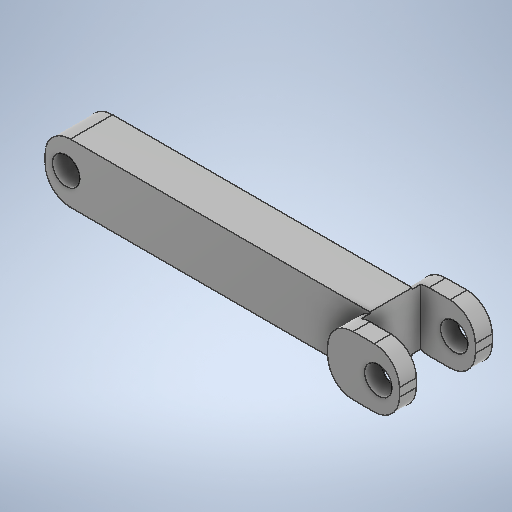
# Autodesk Inventor part: link_arm_1
Saved by Autodesk Inventor 2025 (Build 290162000, 162)
## iProperties
Created: 2025-09-10
Part Number: link_arm_1
Material: 一般
Document SubType Name: Modeling
Designer: sooo1
Density: 1 g/cm^3
Appearance: 滑らか - 標準の灰色
Author: sooo1
Autodesk Inventor part; units mm, degrees
ref_plane "YZ Plane" through (0, 0, 0) normal (1, 0, 0) x (0, 1, 0)
ref_plane "XZ Plane" through (0, 0, 0) normal (0, 1, 0) x (-1, 0, 0)
ref_plane "XY Plane" through (0, 0, 0) normal (0, 0, 1) x (1, 0, 0)
sketch "スケッチ1" plane through (0, 0, 0) normal (0, 0, 1) x (1, 0, 0)
  line L0 (-22.5, 3.5) -> (22.5, 3.5)
  line L1 (22.5, 3.5) -> (22.5, -3.5)
  line L2 (22.5, -3.5) -> (-22.5, -3.5)
  line L3 (-22.5, -3.5) -> (-22.5, 3.5)
  line L4 (-22.5, 3.5) -> (22.5, -3.5) construction
  line L5 (22.5, 3.5) -> (-22.5, -3.5) construction
  line L6 (0, -6.37) -> (0, 6.37) construction
  line L7 (-34.37, 0) -> (34.37, 0) construction
  circle A0 centre (-20, 0) radius 4.55
  line L8 (22.5, -3.5) -> (22.5, 3.5)
  circle A1 centre (20, 0) radius 4.55
  circle A2 centre (-20, 0) radius 1.635
  circle A3 centre (20, 0) radius 1.635
  line L9 (14, 3.5) -> (14, -3.5)
  line L10 (16, 3.5) -> (16, -3.5)
  point P0 (0, 0)
  point P1 (-17.0927, 3.5)
  point P2 (-22.9073, 3.5)
  point P3 (-22.9073, -3.5)
  point P4 (-17.0927, -3.5)
  point P5 (17.0927, 3.5)
  point P6 (17.0927, -3.5)
  point P7 (22.9073, -3.5)
  point P8 (22.9073, 3.5)
  dimension "d1" = 7
  dimension "d2" = 20
  dimension "d3" = 45
  dimension "d4" = 9.1
  dimension "d12" = 3.27
  dimension "d13" = 3.27
  dimension "d14" = 6
  dimension "d15" = 2
  constraints: 18 end point, 5 point on line, 4 centre point, 4 midpoint, 3 perpendicular, 2 coincident, 2 parallel, 1 horizontal, 1 symmetric about line, 1 other
  measures "d1" distance of L2.end L0.start
  measures "d2" distance from line of L6 A0.centre
  measures "d3" distance of L0.start L0.end
  measures "d4" diameter of A0
  measures "d12" diameter of A2
  measures "d13" diameter of A3
  measures "d14" distance from line of L9 A3.centre
  measures "d15" distance between parallel lines of L9 L10
extrude "押し出し1" add sketch "スケッチ1" along normal mid plane 5 contours L9 L2 A0 L0 | L0 L10 A1 L2 L9 | L0 A1 L10 | A0 L2 L3 L0 | L0 L1 L2 A1 L10 | L10 A1 | L10 A1 L2 picked at (-19.7985, 2.8744)
fillet "フィレット1" radius 3 4 edges at (-22.5, 3.5, 0) (-22.5, -3.5, 0) (22.5, -3.5, 0) (22.5, 3.5, 0)
extrude "押し出し3" add sketch "スケッチ1" along normal mid plane 11 contours L0 L10 A1 L2 L9 | L0 A1 L10 | L0 L1 L2 A1 L10 | L10 A1 | L10 A1 L2
extrude "押し出し4" cut sketch "スケッチ1" along normal mid plane 7 contours L0 A1 L10 | L0 L1 L2 A1 L10 | L10 A1 L2
fillet "フィレット2" radius 3 8 edges at (22.5, 3.5, 4.5) (22.5, -3.5, 4.5) (22.5, 3.5, -4.5) (22.5, -3.5, -4.5) (14, 3.5, 4) (14, -3.5, 4) (14, 3.5, -4) (14, -3.5, -4)
